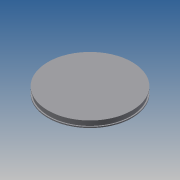
# Autodesk Inventor part: proximal drive pulley
Saved by Autodesk Inventor 2013 (Build 170138000, 138)
## iProperties
Created: 2017-03-06
Part Number: proximal drive pulley
Material: Generic
Document SubType Name: Modeling
Designer: employee
Density: 1 g/cm^3
Author: employee
Autodesk Inventor part; units mm, degrees
ref_plane "YZ Plane" through (0, 0, 0) normal (1, 0, 0) x (0, 1, 0)
ref_plane "XZ Plane" through (0, 0, 0) normal (0, 1, 0) x (-1, 0, 0)
ref_plane "XY Plane" through (0, 0, 0) normal (0, 0, 1) x (1, 0, 0)
sketch "Sketch1" plane through (0, 0, 0) normal (0, 0, 1) x (1, 0, 0)
  circle A0 centre (0, 0) radius 77
  dimension "d0" = 154
  constraints: 1 centre point, 1 coincident
  measures "d0" diameter of A0
extrude "Extrusion1" add sketch "Sketch1" along normal blind 1.5
sketch "Sketch2" plane through (0, 0, 1.5) normal (0, 0, 1) x (1, 0, 0)
  circle A0 centre (0, 0) radius 77 projected
  circle A1 centre (0, 0) radius 75
  dimension "d4" = 150
  constraints: 1 centre point, 1 coincident
  measures "d4" diameter of A1
extrude "Extrusion2" add sketch "Sketch2" along normal blind 7 contours A1
sketch "Sketch3" plane through (0, 0, 8.5) normal (0, 0, 1) x (1, 0, 0)
  circle A0 centre (0, 0) radius 77 projected
extrude "Extrusion3" add sketch "Sketch3" along normal blind 1.5
sketch "Sketch5" plane through (0, 0, 0) normal (0, 0, -1) x (-1, 0, 0)
  circle A0 centre (0, 0) radius 77 projected
  circle A1 centre (0, 0) radius 50
  dimension "d14" = 100
  constraints: 1 centre point, 1 coincident
  measures "d14" diameter of A1
extrude "Extrusion5" add sketch "Sketch5" along normal blind 15 contours A1
sketch "Sketch6" plane through (0, 0, -15) normal (0, 0, -1) x (-1, 0, 0)
  circle A0 centre (0, 0) radius 50 projected
  line L0 (48.4123, 12.5) -> (0, 12.5)
  arc A1 (0, 12.5) -> (0, -12.5) centre (0, 0) ccw
  line L1 (0, -12.5) -> (48.4123, -12.5)
  dimension "d18" = 25
  constraints: 4 end point, 4 point on circle, 2 tangent, 1 centre point, 1 concentric, 1 horizontal
  measures "d18" distance between parallel lines of L1 L0
extrude "Extrusion6" cut sketch "Sketch6" against normal blind 2.5 contours A0 L1 A1 L0 picked at (16.6667, 0)
sketch "Sketch7" plane through (0, 0, 10) normal (0, 0, 1) x (1, 0, 0)
  circle A0 centre (0, 0) radius 77 projected
  circle A1 centre (0, 0) radius 45
  dimension "d22" = 90
  constraints: 1 centre point, 1 coincident
  measures "d22" diameter of A1
extrude "Extrusion7" cut sketch "Sketch7" against normal blind 20 contours A1
sketch "Sketch8" plane through (0, 0, -10) normal (0, 0, 1) x (1, 0, 0)
  circle A0 centre (0, 0) radius 45 projected
  line L0 (0, 35) -> (-105.83, 35)
  line L1 (-105.83, 35) -> (-105.83, -35)
  line L2 (-105.83, -35) -> (0, -35)
  arc A1 (0, -35) -> (0, 35) centre (0, 0) ccw
  dimension "d26" = 70
  constraints: 6 end point, 2 point on circle, 2 tangent, 1 centre point, 1 coincident, 1 horizontal, 1 parallel, 1 perpendicular
  measures "d26" distance between parallel lines of L2 L0
extrude "Extrusion8" cut sketch "Sketch8" along normal up to surface (10 mm away) contours L0 A1 L2 A0 | A0 L2 L1 L0 picked at (-14.9265, 1.4828)
body "Solid1"
